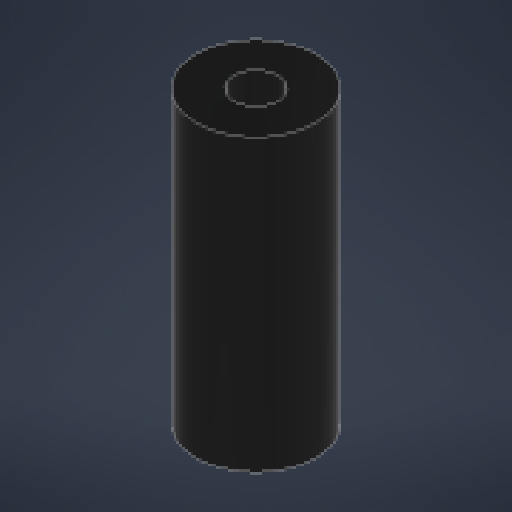
# Autodesk Inventor part: grapple-pivot-shaft
Saved by Autodesk Inventor 2025.1 (Build 291241020, 241B)
## iProperties
Created: 2025-03-18
Part Number: grapple-pivot-shaft
Material: ABS Plastic
Document SubType Name: Modeling
Designer: mathe
Density: 1.06 g/cm^3
Appearance: Smooth - White
Author: mathe
Autodesk Inventor part; units mm, degrees
ref_plane "YZ Plane" through (0, 0, 0) normal (1, 0, 0) x (0, 1, 0)
ref_plane "XZ Plane" through (0, 0, 0) normal (0, 1, 0) x (-1, 0, 0)
ref_plane "XY Plane" through (0, 0, 0) normal (0, 0, 1) x (1, 0, 0)
sketch "Sketch1" plane through (0, 0, 0) normal (0, 1, 0) x (-1, 0, 0)
  circle A0 centre (0, 0) radius 6.858
  dimension "d0" = 13.716
  constraints: 1 centre point, 1 coincident
  measures "d0" diameter of A0
extrude "Extrusion1" add sketch "Sketch1" along normal blind 33.3375
hole "Hole1" at (0, 0, 0) direction (0, 1, 0) diameter 5.1 end through all
body "Solid1"
